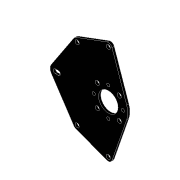
# Autodesk Inventor part: steel_plate7
Saved by Autodesk Inventor 2022 (Build 260153000, 153)
## iProperties
Created: 2021-08-14
Part Number: steel_plate7
Material: 鋼、炭素鋼
Document SubType Name: Sheet Metal
Designer: yuta0
Density: 7.85 g/cm^3
Sheet Metal Rule: Default_mm
Appearance: 滑らか - 黒
Author: yuta0
Autodesk Inventor part; units mm, degrees
ref_plane "YZ Plane" through (0, 0, 0) normal (1, 0, 0) x (0, 1, 0)
ref_plane "XZ Plane" through (0, 0, 0) normal (0, 1, 0) x (-1, 0, 0)
ref_plane "XY Plane" through (0, 0, 0) normal (0, 0, 1) x (1, 0, 0)
sketch "スケッチ1" plane through (0, 0, 0) normal (0, 0, 1) x (1, 0, 0)
  circle A0 centre (0, 0) radius 42.5 construction
  arc A1 (71.9037, -6.5306) -> (71.9037, 6.5306) centre (53, 0) ccw
  circle A2 centre (53, 0) radius 49 construction
  arc A3 (-5.838, 3.8623) -> (-5.838, -3.8623) centre (0, 0) ccw
  arc A4 (19.4901, 40.7594) -> (17.317, 38.812) centre (20.8892, 37.0121) ccw
  arc A5 (17.317, -38.812) -> (19.4901, -40.7594) centre (20.8892, -37.0121) ccw
  arc A6 (56.7807, 50.3061) -> (51.601, 52.7474) centre (53, 49) ccw
  arc A7 (51.601, -52.7474) -> (56.7807, -50.3061) centre (53, -49) ccw
  line L0 (19.4901, 40.7594) -> (51.601, 52.7474)
  line L1 (56.7807, 50.3061) -> (71.9037, 6.5306)
  line L2 (71.9037, -6.5306) -> (56.7807, -50.3061)
  line L3 (51.601, -52.7474) -> (19.4901, -40.7594)
  line L4 (17.5531, -39.2191) -> (-5.838, -3.8623)
  line L5 (-5.838, 3.8623) -> (17.5531, 39.2191)
  dimension "d0" = 53
  dimension "d1" = 40
  dimension "d2" = 98
  dimension "d3" = 85
  dimension "d4" = 14
  dimension "d5" = 8
  dimension "d6" = 8
  dimension "d7" = 8
  dimension "d8" = 8
  measures "d0" distance of A0.centre A1.centre
  measures "d1" diameter of A1
  measures "d2" diameter of A2
  measures "d3" diameter of A0
  measures "d4" diameter of A3
  measures "d5" diameter of A4
  measures "d6" diameter of A5
  measures "d7" diameter of A6
  measures "d8" diameter of A7
extrude "プレート1" add sketch "スケッチ1" along normal blind 2.3
sketch "スケッチ2" plane through (0, 0, 2.3) normal (0, 0, 1) x (1, 0, 0)
  arc A0 (71.9037, -6.5306) -> (71.9037, 6.5306) centre (53, 0) ccw projected
  line L0 (56.7807, 50.3061) -> (71.9037, 6.5306) projected
  arc A1 (56.7807, 50.3061) -> (51.601, 52.7474) centre (53, 49) ccw projected
  line L1 (19.4901, 40.7594) -> (51.601, 52.7474) projected
  arc A2 (19.4901, 40.7594) -> (17.5531, 39.2191) centre (20.8892, 37.0121) ccw projected
  line L2 (-5.838, 3.8623) -> (17.5531, 39.2191) projected
  arc A3 (-5.838, 3.8623) -> (-5.838, -3.8623) centre (0, 0) ccw projected
  line L3 (17.5531, -39.2191) -> (-5.838, -3.8623) projected
  arc A4 (17.5531, -39.2191) -> (19.4901, -40.7594) centre (20.8892, -37.0121) ccw projected
  line L4 (51.601, -52.7474) -> (19.4901, -40.7594) projected
  arc A5 (51.601, -52.7474) -> (56.7807, -50.3061) centre (53, -49) ccw projected
  line L5 (71.9037, -6.5306) -> (56.7807, -50.3061) projected
hole "穴1" at (53, 49, 2.3) at (53, -49, 2.3) at (20.8892, 37.0121, 2.3) at (20.8892, -37.0121, 2.3) direction (0, 0, -1) diameter 4.3 depth 2.3 clearance for "Flat Head Machine Screw" size "M4" standard "Ansi Metric M Profile"
sketch "スケッチ3" plane through (0, 0, 2.3) normal (0, 0, 1) x (1, 0, 0)
  arc A0 (71.9037, -6.5306) -> (71.9037, 6.5306) centre (53, 0) ccw projected
  circle A1 centre (53, 0) radius 10
  point P0 (0, 0)
  dimension "d17" = 20
  constraints: 1 centre point, 1 coincident
  measures "d17" diameter of A1
extrude "押し出し1" cut sketch "スケッチ3" against normal blind 10
sketch "スケッチ4" plane through (0, 0, 2.3) normal (0, 0, 1) x (1, 0, 0)
  arc A0 (71.9037, -6.5306) -> (71.9037, 6.5306) centre (53, 0) ccw projected
  circle A1 centre (53, 0) radius 15
  point P0 (0, 0)
  point P1 (38, 0)
  point P2 (53, -15)
  point P3 (68, 0)
  point P4 (53, 15)
  dimension "d20" = 30
  dimension "d23" = 360
  constraints: 1 coincident, 1 horizontal alignment, 7 other
hole "穴2" at (38, 0, 2.3) at (53, -15, 2.3) at (68, 0, 2.3) at (53, 15, 2.3) direction (0, 0, -1) diameter 3.2 depth 2.3 clearance for "Flat Head Machine Screw" size "M3" standard "Ansi Metric M Profile"
sketch "スケッチ5" plane through (0, 0, 2.3) normal (0, 0, 1) x (1, 0, 0)
  arc A0 (71.9037, -6.5306) -> (71.9037, 6.5306) centre (53, 0) ccw projected
  circle A1 centre (53, 0) radius 16
  point P0 (0, 0)
  point P1 (41.6863, 11.3137)
  point P2 (41.6863, -11.3137)
  point P3 (64.3137, -11.3137)
  point P4 (64.3137, 11.3137)
  dimension "d32" = 32
  dimension "d35" = 360
  constraints: 1 coincident, 1 horizontal alignment, 8 other
hole "穴3" at (41.6863, 11.3137, 2.3) at (41.6863, -11.3137, 2.3) at (64.3137, -11.3137, 2.3) at (64.3137, 11.3137, 2.3) direction (0, 0, -1) diameter 4.3 depth 2.3 clearance for "Flat Head Machine Screw" size "M4" standard "Ansi Metric M Profile"
sketch "スケッチ6" plane through (0, 0, 2.3) normal (0, 0, 1) x (1, 0, 0)
  arc A0 (-5.838, 3.8623) -> (-5.838, -3.8623) centre (0, 0) ccw projected
hole "穴4" at (0, 0, 2.3) direction (0, 0, -1) diameter 4.3 depth 2.3 clearance for "Flat Head Machine Screw" size "M4" standard "Ansi Metric M Profile"
sketch "スケッチ7" plane through (0, 0, 2.3) normal (0, 0, 1) x (1, 0, 0)
  line L0 (-1.5, 0) -> (1.5, 0) construction
  line L1 (-1.5, -2.15) -> (1.5, -2.15)
  line L2 (1.5, 2.15) -> (-1.5, 2.15)
  arc A0 (-1.5, 2.15) -> (-1.5, -2.15) centre (-1.5, 0) ccw
  arc A1 (1.5, -2.15) -> (1.5, 2.15) centre (1.5, 0) ccw
  circle A2 centre (0, 0) radius 2.15 projected
  point P0 (0, 2.15)
  point P1 (0, -2.15)
  dimension "d51" = 3
  constraints: 8 end point, 5 tangent, 4 point on circle, 2 centre point, 1 horizontal, 1 midpoint, 1 parallel
  measures "d51" distance of L1.start L1.end
extrude "押し出し2" cut sketch "スケッチ7" against normal blind 10
equation "\"d15\" = Thickness"
equation "\"d30\" = Thickness"
equation "\"d42\" = Thickness"
equation "\"d49\" = Thickness"
equation "\"d9\" = Thickness"
equation "\"BendRadius\" = Thickness"
equation "\"BendReliefWidth\" = Thickness"
equation "\"BendReliefDepth\" = 0.5 * Thickness"
equation "\"CornerReliefSize\" = 4 * Thickness"
equation "\"MinimumRemnant\" = 2 * Thickness"
equation "\"TransitionRadius\" = BendRadius"
equation "\"JacobiRadiusSize\" = BendRadius"
equation "\"GapSize\" = Thickness"
equation "\"Thickness\" = 2.3"
